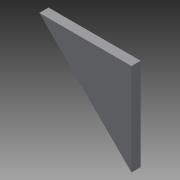
# Autodesk Inventor part: wspornik
Saved by Autodesk Inventor 2015 (Build 190159000, 159)
## iProperties
Created: 2015-05-04
Part Number: wspornik
Material: Ogólny
Document SubType Name: Modeling
Designer: Kuba
Density: 1 g/cm^3
Appearance: Domyślna
Author: Kuba
Autodesk Inventor part; units mm, degrees
ref_plane "YZ Plane" through (0, 0, 0) normal (1, 0, 0) x (0, 1, 0)
ref_plane "XZ Plane" through (0, 0, 0) normal (0, 1, 0) x (-1, 0, 0)
ref_plane "XY Plane" through (0, 0, 0) normal (0, 0, 1) x (1, 0, 0)
sketch "Szkic1" plane through (0, 0, 0) normal (0, 1, 0) x (-1, 0, 0)
  line L0 (0, 0) -> (20, 0)
  line L1 (0, -20) -> (0, 0)
  line L2 (20, 0) -> (0, -20)
  dimension "d2" = 20
  dimension "d3" = 20
  dimension "d4" = 45
  constraints: 6 end point, 1 horizontal
  measures "d2" distance of L0.start L0.end
  measures "d3" distance of L1.start L0.start
  measures "d4" angle of L1 L2
extrude "Wyciągnięcie proste1" add sketch "Szkic1" along normal blind 2
